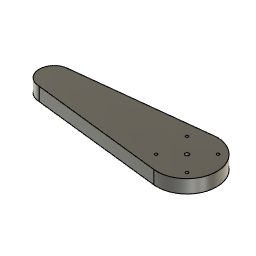
3-braco-2 v2 (Autodesk Fusion 360 design; units mm, degrees)
Autodesk Fusion 360 part; units mm, degrees
sketch "Sketch1" plane through (0, 0, 0) normal (0, 0, 1) x (1, 0, 0)
  circle A0 centre (-74.4665, 27.0941) radius 22.5
  line L0 (-74.4665, 27.0941) -> (-74.4665, 117.7427) construction
  line L1 (125.5335, 27.0941) -> (125.5335, 120) construction
  line L2 (-74.4665, 27.0941) -> (124.443, 27.0941) construction
  line L3 (25.5335, 130) -> (25.5335, -85.9983) construction
  circle A1 centre (125.5335, 27.0941) radius 45
  line L4 (-74.4665, 49.5941) -> (125.5335, 72.0941)
  line L5 (-74.3843, 4.5942) -> (120.4363, -17.6163)
  circle A2 centre (125.5335, 27.3791) radius 3
  circle A3 centre (102.199, 50.7137) radius 1.665
  circle A4 centre (102.199, 4.0446) radius 1.665
  circle A5 centre (149.443, 3.4697) radius 1.665
  circle A6 centre (148.868, 50.7137) radius 1.665
  line L6 (102.199, 50.7137) -> (149.443, 50.7137)
  line L7 (149.443, 50.7137) -> (149.443, 3.4697)
  line L8 (149.443, 3.4697) -> (102.199, 3.4697)
  line L9 (102.199, 3.4697) -> (102.199, 50.7137)
  point P0 (125.5335, 27.3791)
  point P1 (125.5335, 27.3791)
  dimension "d1" = 45
  dimension "d3" = 200
  dimension "d4" = 100
  dimension "d6" = 33
  dimension "d9" = 6
  dimension "d10" = 3.33
  dimension "d11" = 3.33
  dimension "d12" = 3.33
  dimension "d13" = 3.33
  dimension "d14" = 90
  dimension "d15" = 47.244
  dimension "d16" = 47.244
  constraint coincident A0.centre L0.start
  constraint vertical L0
  constraint vertical L1
  constraint perpendicular L0 L2
  constraint vertical L3
  constraint coincident P1 P0
  constraint coincident L1.start A1.centre
  constraint coincident A0 L4.start
  constraint coincident L0 L4.start
  constraint coincident A1 L4.end
  constraint coincident L1 L4.end
  constraint coincident A0 L5.start
  constraint coincident A1 L5.end
  constraint tangent A1 L5
  constraint horizontal L6
  constraint vertical L7
  constraint horizontal L8
  constraint vertical L9
  constraint coincident A5.centre L7.end
  constraint coincident A3.centre L6.start
  measures "d1" diameter of A0
  measures "d3" distance of A0.centre L1.start
  measures "d4" distance of L0 L3
  measures "d6" distance of P1 A6.centre
  measures "d9" diameter of A2
  measures "d10" diameter of A3
  measures "d11" diameter of A4
  measures "d12" diameter of A5
  measures "d13" diameter of A6
  measures "d14" diameter of A1
  measures "d15" distance of A3.centre L6.end
  measures "d16" distance of L6.end A5.centre
extrude "Extrude1" add sketch "Sketch1" against normal blind 20 contours A0 | A0 A1 L4 L5 | A1 L4 | A2 | A3 L6 L9 | A3 A4 A5 A6 L6 L7 L8 L9 | A3 L6 L9 | A6 L6 L7 | A6 L6 L7 | A4 L8 L9 | A4 L8 L9 | A5 L7 L8 | A5 L7 L8 picked at (94.9797, 27.5619)
hole "Hole1" at (102.199, 50.7137, 0) at (102.199, 4.0446, 0) at (149.443, 3.4697, 0) at (148.868, 50.7137, 0) direction (0, 0, -1) diameter 4 depth 10 tip angle 118
extrude "Extrude2" cut sketch "Sketch1" against normal blind 6 contours A2
